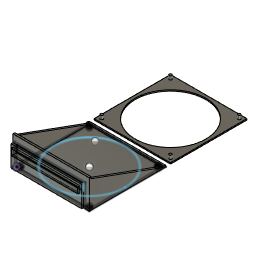
MSI Pulse76 CPU Repalcement v2 (Autodesk Fusion 360 design; units mm, degrees)
Autodesk Fusion 360 part; units mm, degrees
sketch "Sketch1" plane through (0, 0, 0) normal (0, 0, 1) x (1, 0, 0)
  line L0 (0, 0) -> (76, 0)
  line L1 (76, 0) -> (76, 76)
  line L2 (76, 76) -> (0, 76)
  line L3 (0, 76) -> (0, 0)
  circle A0 centre (2, 74) radius 2
  circle A1 centre (74, 74) radius 2
  circle A2 centre (74, 2) radius 2
  circle A3 centre (2, 2) radius 2
  line L4 (-2, -2) -> (78, -2)
  line L5 (78, -2) -> (78, 78)
  line L6 (78, 78) -> (-2, 78)
  line L7 (-2, 78) -> (-2, -2)
  circle A4 centre (38, 38) radius 38
  circle A5 centre (38, 38) radius 37
  circle A6 centre (2, 74) radius 1.4
  circle A7 centre (74, 74) radius 1.4
  circle A8 centre (74, 2) radius 1.4
  circle A9 centre (2, 2) radius 1.4
  point P0 (17.79, 64.2008)
  dimension "d1" = 76
  dimension "d2" = 76
  dimension "d3" = 4
  dimension "d4" = 4
  dimension "d5" = 4
  dimension "d6" = 4
  dimension "d7" = 2
  dimension "d8" = -1
  dimension "d11" = -0.6
  dimension "d12" = -0.6
  dimension "d13" = -0.6
  dimension "d14" = -0.6
  constraint horizontal L0
  constraint vertical L1
  constraint horizontal L2
  constraint vertical L3
  constraint coincident L0.start L3.end
  constraint tangent L2 A0
  constraint tangent L3 A0
  constraint tangent L2 A1
  constraint tangent L1 A1
  constraint tangent L1 A2
  constraint tangent L0 A2
  constraint tangent L0 A3
  constraint tangent L3 A3
  constraint tangent L2 A4
  measures "d1" distance of L0.start L0.end
  measures "d2" distance of L0.start L2.end
  measures "d3" diameter of A0
  measures "d4" diameter of A1
  measures "d5" diameter of A2
  measures "d6" diameter of A3
extrude "Extrude1" add sketch "Sketch1" along normal blind 1.2 contours L0 L3 A3 | L0 L3 A3 A4 | A3 | L0 L1 A2 A4 | A4 | L2 L3 A0 A4 | L0 L1 A2 | A2 | L1 L2 A1 A4 | L2 L3 A0 | A0 | L1 L2 A1 | A1 | L4 L5 L6 L7 | A6 | A7 | A8 | A9 makes body 1
extrude "Extrude2" add sketch "Sketch1" along normal blind 5 contours A6 | A7 | A8 | A9 bodies 1
move_body "Move1" bodies 1 to x (1, 0, 0) y (0, 0.996195, -0.087156) z (0, 0.087156, 0.996195) at (0, 0.2968, 6.7981)
sketch "Sketch2" plane through (0, 0, 0) normal (0, 1, 0) x (1, 0, 0)
  line L0 (0, 0) -> (70, 0)
  line L1 (70, 0) -> (70, -20)
  line L2 (70, -20) -> (0, -20)
  line L3 (0, -20) -> (0, 0)
  line L4 (0, -20) -> (70, -20)
  line L5 (70, -20) -> (70, -13)
  line L6 (70, -13) -> (0, -13)
  line L7 (0, -13) -> (0, -20)
  line L8 (-2, -22) -> (-2, 0)
  line L9 (72, 0) -> (72, -22)
  line L10 (72, -22) -> (-2, -22)
  line L11 (-2, 0) -> (0, 0)
  line L12 (70, 0) -> (72, 0)
  line L13 (0, -13) -> (70, -13)
  line L14 (70, -13) -> (70, -20)
  line L15 (70, -20) -> (0, -20)
  line L16 (0, -20) -> (0, -13)
  line L17 (0.5, -19.5) -> (0.5, -13.5)
  line L18 (69.5, -13.5) -> (0.5, -13.5)
  line L19 (69.5, -19.5) -> (69.5, -13.5)
  line L20 (69.5, -19.5) -> (0.5, -19.5)
  dimension "d18" = 70
  dimension "d19" = 20
  dimension "d20" = 7
  dimension "d25" = 0.5
  constraint horizontal L0
  constraint vertical L1
  constraint horizontal L2
  constraint vertical L3
  constraint coincident L0.start L3.end
  constraint horizontal L4
  constraint vertical L5
  constraint horizontal L6
  constraint vertical L7
  constraint perpendicular L3 L11
  constraint perpendicular L9 L12
  constraint horizontal L13
  constraint vertical L14
  constraint horizontal L15
  constraint vertical L16
  measures "d18" distance of L0.start L0.end
  measures "d19" distance of L0.start L2.end
  measures "d20" distance of L2.end L6.end
extrude "Extrude3" add sketch "Sketch2" against normal blind 4 separate body contours L0 L1 L3 L6 L13 | L1 L2 L3 L4 L5 L7 L8 L9 L10 L11 L12 L14 L15 L16 makes body 2
move_body "Move2" bodies 1 to x (1, 0, 0) y (0, 0.965926, -0.258819) z (0, 0.258819, 0.965926) at (0, 2.6578, 20.1879)
extrude "Extrude4" add sketch "Sketch2" against normal blind 6 contours L1 L2 L3 L4 L5 L6 L7 L13 L14 L15 L16 bodies 2
sketch "Sketch3" plane through (0, 0, 0) normal (1, 0, 0) x (0, 1, 0)
  line L0 (0, 0) -> (82.4686, 0)
  line L1 (82.4686, 0) -> (82.4686, 33.3706)
  line L2 (82.4686, 33.3706) -> (0, 33.3706)
  line L3 (0, 33.3706) -> (0, 0)
  line L4 (78, 0) -> (0, 29)
  constraint horizontal L0
  constraint vertical L1
  constraint horizontal L2
  constraint vertical L3
  constraint coincident L0.start L3.end
  constraint coincident L0 L4.start
  constraint coincident L3 L4.end
extrude "Extrude5" add sketch "Sketch1" along normal blind 30 separate body contours L4 L5 L6 L7 makes body 3
extrude "Extrude6" cut sketch "Sketch3" along normal blind 108 and the other way blind 15 contours L0 L1 L2 L3 L4 bodies 3
move_body "Move3" bodies 1 to x (1, 0, 0) y (0, 1, 0) z (0, 0, 1) at (0, -3, 1)
extrude "Extrude7" add 1 faces at (51.3333, 75.2736, 1.7518) along direction (0, 0.939693, -0.34202) blind 3 separate body on bodies 1 makes body 4
extrude "Extrude8" cut sketch "Sketch2" against normal blind 23 contours L17 L18 L19 L20 bodies 3
combine "Combine1" operation cut target body 3 tool bodies 1 keep tools
move_body "Move4" bodies 1 to x (1, 0, 0) y (0, 1, 0) z (0, 0, 1) at (0, 0, 9)
extrude "Extrude9" add 1 faces at (50.6667, 76, 0.2479) along direction (0, -1, 0) blind 78 on bodies 3 bodies 3 2 4
draft "Draft1" angle -5 neutral plane through (0, -4, 0) pull (0, -1, 0) 1 faces at (46.5, -2, 13.5) on bodies 3
draft "Draft2" angle 10 neutral plane through (0, -4, 0) pull (0, -1, 0) 1 faces at (46.6667, -4.6667, 13) on bodies 3
copy_body "CopyPasteBodies1" bodies 1 makes body 5
move_body "Move5" bodies 5 to x (1, 0, 0) y (0, 1, 0) z (0, 0, 1) at (0, 90, 0)
move_body "Move6" bodies 5 to x (1, 0, 0) y (0, 0.939693, 0.34202) z (0, -0.34202, 0.939693) at (0, 13.3709, -55.8302)
move_body "Move7" bodies 5 to x (1, 0, 0) y (0, 1, 0) z (0, 0, 1) at (0, -87, -10)
move_body "Move8" bodies 5 to x (1, 0, 0) y (0, 1, 0) z (0, 0, 1) at (0, 85, 0)
hidden bodies 1
